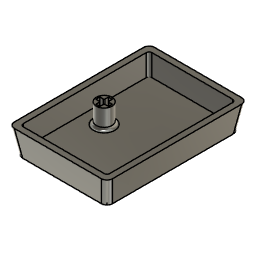
keycaps_tiapad_lcd_f1_f4 (Autodesk Fusion 360 design; units mm, degrees)
Autodesk Fusion 360 part; units mm, degrees
sketch "Schizzo1" plane through (0, 0, 0) normal (0, 0, 1) x (1, 0, 0) in component "keycap"
  circle A0 centre (0, 0) radius 2.8
  line L0 (2.25, 2.25) -> (-2.25, 2.25) construction
  line L1 (-2.25, 2.25) -> (-2.25, -2.25) construction
  line L2 (-2.25, -2.25) -> (2.25, -2.25) construction
  line L3 (2.25, -2.25) -> (2.25, 2.25) construction
  line L4 (2.25, 2.25) -> (-2.25, -2.25) construction
  line L5 (-2.25, 2.25) -> (2.25, -2.25) construction
  line L6 (0.685, 2.2283) -> (-0.685, 2.2283)
  line L7 (-0.685, 2.2283) -> (-0.685, -2.2283)
  line L8 (-0.685, -2.2283) -> (0.685, -2.2283)
  line L9 (0.685, -2.2283) -> (0.685, 2.2283)
  line L10 (0.685, 2.2283) -> (-0.685, -2.2283) construction
  line L11 (-0.685, 2.2283) -> (0.685, -2.2283) construction
  line L12 (2.2283, 0.685) -> (-2.2283, 0.685)
  line L13 (-2.2283, 0.685) -> (-2.2283, -0.685)
  line L14 (-2.2283, -0.685) -> (2.2283, -0.685)
  line L15 (2.2283, -0.685) -> (2.2283, 0.685)
  line L16 (2.2283, 0.685) -> (-2.2283, -0.685) construction
  line L17 (-2.2283, 0.685) -> (2.2283, -0.685) construction
  dimension "d7" = 5.6
  dimension "d8" = 4.5
  dimension "d9" = 4.5
  dimension "d10" = 1.37
  dimension "d11" = 1.37
  constraint coincident A0.centre origin
  constraint horizontal L0
  constraint perpendicular L0 L1
  constraint parallel L0 L2
  constraint parallel L1 L3
  constraint coincident L4 A0.centre
  constraint coincident L5 A0.centre
  constraint horizontal L6
  constraint perpendicular L6 L7
  constraint parallel L6 L8
  constraint parallel L7 L9
  constraint coincident L10 A0.centre
  constraint coincident L11 A0.centre
  constraint horizontal L12
  constraint perpendicular L12 L13
  constraint parallel L12 L14
  constraint parallel L13 L15
  constraint coincident L16 A0.centre
  constraint coincident L17 A0.centre
  measures "d7" diameter of A0
  measures "d8" distance of L1.end L2.end
  measures "d9" distance of L0.end L1.end
  measures "d10" distance of L7.end L8.end
  measures "d11" distance of L12.end L13.end
extrude "Estrusione1" add sketch "Schizzo1" along normal blind 8.45 makes body 1 in component "keycap"
fillet "Raccordo1" radius 0.3 4 edges at (-0.685, 0.685, 4.225) (0.685, 0.685, 4.225) (0.685, -0.685, 4.225) (-0.685, -0.685, 4.225) on bodies 1 in component "keycap"
sketch "Schizzo6" plane through (0, 0, 0) normal (0, 0, -1) x (1, 0, 0)
  arc A0 (-0.985, 0.685) -> (-0.685, 0.985) centre (-0.985, 0.985) ccw
  line L0 (-0.685, 0.985) -> (-0.685, 2.2283)
  line L1 (-0.685, 2.2283) -> (0.685, 2.2283)
  line L2 (0.685, 2.2283) -> (0.685, 0.985)
  arc A1 (0.685, 0.985) -> (0.985, 0.685) centre (0.985, 0.985) ccw
  line L3 (0.985, 0.685) -> (2.2283, 0.685)
  line L4 (2.2283, 0.685) -> (2.2283, -0.685)
  line L5 (2.2283, -0.685) -> (0.985, -0.685)
  arc A2 (0.985, -0.685) -> (0.685, -0.985) centre (0.985, -0.985) ccw
  line L6 (0.685, -0.985) -> (0.685, -2.2283)
  line L7 (0.685, -2.2283) -> (-0.685, -2.2283)
  line L8 (-0.685, -2.2283) -> (-0.685, -0.985)
  arc A3 (-0.685, -0.985) -> (-0.985, -0.685) centre (-0.985, -0.985) ccw
  line L9 (-0.985, -0.685) -> (-2.2283, -0.685)
  line L10 (-2.2283, -0.685) -> (-2.2283, 0.685)
  line L11 (-2.2283, 0.685) -> (-0.985, 0.685)
  circle A4 centre (0, 0) radius 2.8
  line L12 (-7, -7) -> (7, -7)
  line L13 (7, -7) -> (7, 7)
  line L14 (7, 7) -> (-7, 7)
  line L15 (-7, 7) -> (-7, -7)
  line L16 (-7, -7) -> (7, 7) construction
  line L17 (7, -7) -> (-7, 7) construction
  line L18 (9.1, -9.1) -> (-9.1, -9.1)
  line L19 (-9.1, -9.1) -> (-9.1, 9.1)
  line L20 (-9.1, 9.1) -> (9.1, 9.1)
  line L21 (9.1, 9.1) -> (9.1, -9.1)
  line L22 (9.1, -9.1) -> (-9.1, 9.1) construction
  line L23 (-9.1, -9.1) -> (9.1, 9.1) construction
  line L24 (7.6, 7.6) -> (7.6, -7.6)
  line L25 (7.6, -7.6) -> (-7.6, -7.6)
  line L26 (-7.6, -7.6) -> (-7.6, 7.6)
  line L27 (-7.6, 7.6) -> (7.6, 7.6)
  dimension "d37" = 14
  dimension "d38" = 14
  dimension "d42" = 18.2
  dimension "d43" = 18.2
  dimension "d44" = 1.5
  constraint horizontal L12
  constraint perpendicular L12 L13
  constraint parallel L12 L14
  constraint parallel L13 L15
  constraint coincident L16 A4.centre
  constraint coincident L17 A4.centre
  constraint coincident A4.centre origin
  constraint horizontal L18
  constraint perpendicular L18 L19
  constraint parallel L18 L20
  constraint parallel L19 L21
  constraint coincident L22 A4.centre
  constraint coincident L23 A4.centre
  measures "d37" distance of L13.end L14.end
  measures "d38" distance of L12.end L13.end
  measures "d42" distance of L19.end L20.end
  measures "d43" distance of L18.end L19.end
sketch "Schizzo13" plane through (0, 0, 0) normal (0, 0, -1) x (1, 0, 0)
  arc A0 (-0.985, 0.685) -> (-0.685, 0.985) centre (-0.985, 0.985) ccw
  line L0 (-0.685, 0.985) -> (-0.685, 2.2283)
  line L1 (-0.685, 2.2283) -> (0.685, 2.2283)
  line L2 (0.685, 2.2283) -> (0.685, 0.985)
  arc A1 (0.685, 0.985) -> (0.985, 0.685) centre (0.985, 0.985) ccw
  line L3 (0.985, 0.685) -> (2.2283, 0.685)
  line L4 (2.2283, 0.685) -> (2.2283, -0.685)
  line L5 (2.2283, -0.685) -> (0.985, -0.685)
  arc A2 (0.985, -0.685) -> (0.685, -0.985) centre (0.985, -0.985) ccw
  line L6 (0.685, -0.985) -> (0.685, -2.2283)
  line L7 (0.685, -2.2283) -> (-0.685, -2.2283)
  line L8 (-0.685, -2.2283) -> (-0.685, -0.985)
  arc A3 (-0.685, -0.985) -> (-0.985, -0.685) centre (-0.985, -0.985) ccw
  line L9 (-0.985, -0.685) -> (-2.2283, -0.685)
  line L10 (-2.2283, -0.685) -> (-2.2283, 0.685)
  line L11 (-2.2283, 0.685) -> (-0.985, 0.685)
  circle A4 centre (0, 0) radius 2.8
  line L12 (0, 0) -> (-9, 0) construction
  line L13 (-9, 0) -> (-9, 25) construction
  line L14 (-9, 25) -> (26, 25)
  line L15 (26, 25) -> (26, -25)
  line L16 (26, -25) -> (-9, -25)
  line L17 (-9, -25) -> (-9, 25)
  line L18 (24.5, 23.5) -> (24.5, -23.5)
  line L19 (24.5, -23.5) -> (-7.5, -23.5)
  line L20 (-7.5, -23.5) -> (-7.5, 23.5)
  line L21 (-7.5, 23.5) -> (24.5, 23.5)
  line L22 (23.9, 22.9) -> (23.9, -22.9)
  line L23 (23.9, -22.9) -> (-6.9, -22.9)
  line L24 (-6.9, -22.9) -> (-6.9, 22.9)
  line L25 (-6.9, 22.9) -> (23.9, 22.9)
  dimension "d65" = 9
  dimension "d66" = 25
  dimension "d67" = 35
  dimension "d68" = 50
  dimension "d69" = 1.5
  dimension "d70" = 2.1
  constraint coincident A4.centre L12.start
  constraint parallel L3 L12
  constraint perpendicular L12 L13
  constraint horizontal L14
  constraint vertical L15
  constraint horizontal L16
  constraint vertical L17
  measures "d65" distance of A4.centre L12.end
  measures "d66" distance of L12.end L13.end
  measures "d67" distance of L13.end L14.end
  measures "d68" distance of L13.end L16.end
extrude "Estrusione5" add sketch "Schizzo13" against normal blind 9.2 separate body contours L14 L15 L16 L17 | L18 L19 L20 L21 makes body 2
extrude "Estrusione6" [suppressed]
extrude "Estrusione8" add sketch "Schizzo13" against normal blind 1.5 contours A0 L0 L1 L2 A1 L3 L4 L5 A2 L6 L7 L8 A3 L9 L10 L11 | A4 | L22 L23 L24 L25 bodies 1 in component "keycap"
sketch "Schizzo14" plane through (0, -25, 0) normal (0, -1, 0) x (1, 0, 0)
  line L0 (-9, 0) -> (26, 0)
  line L1 (26, 0) -> (26, 9.2)
  line L2 (26, 9.2) -> (-9, 9.2)
  line L3 (-9, 9.2) -> (-9, 0)
  line L4 (-9, 9.2) -> (-7.5, 0)
  line L5 (26, 9.2) -> (24.5, 0)
  point P0 (-7.5, 0)
  point P1 (24.5, 0)
  constraint coincident L2.end L3.start
  constraint coincident P0 L4.end
  constraint coincident L1.end L2.start
  constraint coincident P1 L5.end
sketch "Schizzo15" plane through (26, 0, 0) normal (1, 0, 0) x (0, 1, 0)
  line L0 (-25, 0) -> (25, 0)
  line L1 (25, 0) -> (25, 9.2)
  line L2 (25, 9.2) -> (-25, 9.2)
  line L3 (-25, 9.2) -> (-25, 0)
  line L4 (-25, 9.2) -> (-23.5, 0)
  line L5 (25, 9.2) -> (23.5, 0)
  point P0 (-23.5, 0)
  point P1 (23.5, 0)
  constraint coincident L2.end L3.start
  constraint coincident P0 L4.end
  constraint coincident L1.end L2.start
  constraint coincident P1 L5.end
extrude "Estrusione7" cut sketch "Schizzo14" against normal through all contours L0 L3 L4 | L0 L1 L5 bodies 2
extrude "Estrusione8'" cut sketch "Schizzo15" against normal through all contours L0 L3 L4 | L0 L1 L5 bodies 2
fillet "Raccordo4" radius 1 1 edges at (-2.6105, -1.0125, 1.5) on bodies 1 in component "keycap"
fillet "Raccordo5" radius 0.5 1 faces at (0.2528, 0.2427, 1.5) on bodies 1 in component "keycap"
fillet "Raccordo4'" radius 1 4 edges at (-6.9, 22.9, 4.6) (23.9, 22.9, 4.6) (23.9, -22.9, 4.6) (-6.9, -22.9, 4.6) on bodies 2
fillet "Raccordo5'" radius 2 4 edges at (25.25, 24.25, 4.6) (-8.25, 24.25, 4.6) (-8.25, -24.25, 4.6) (25.25, -24.25, 4.6) on bodies 2
component "keycap" placed x (1, 0, 0) y (0, 1, 0) z (0, 0, 1) at (0, 0, 0)
component "keycap_1" placed x (1, 0, 0) y (0, 1, 0) z (0, 0, 1) at (0, 0, 0)
equation "tol = 0.2 mm"
equation "keystem_height = 3.6 mm"
equation "keystem_cross_lenght = 4.1 mm + tol * 2"
equation "keystem_cross_armwidth = 1.17 mm + tol"
equation "keystem_angle_curvature = 0.3 mm"
equation "shaft_diameter = 5.4 mm + tol"
equation "d7 = shaft_diameter"
equation "d8 = keystem_cross_lenght"
equation "d9 = keystem_cross_lenght"
equation "d10 = keystem_cross_armwidth"
equation "d11 = keystem_cross_armwidth"
equation "d12 = keycap_height - keycap_plasticthickness / 2"
equation "d15 = keystem_angle_curvature"
equation "keycap_side_bottom = 18.2 mm"
equation "keycap_height = 9.2 mm"
equation "keycap_plasticthickness = 1.5 mm"
equation "keycap_side_top = 14 mm"
equation "d37 = keycap_side_top"
equation "d38 = keycap_side_top"
equation "d42 = keycap_side_bottom"
equation "d43 = keycap_side_bottom"
equation "d44 = keycap_plasticthickness"
equation "keycap_f1_f4_side_short = 35 mm"
equation "keycap_f1_f4_side_long = 50 mm"
equation "keycap_f1_f4_dist_from_side_short = 9 mm"
equation "keycap_f1_f4_dist_from_top = keycap_f1_f4_side_long / 2"
equation "d65 = keycap_f1_f4_dist_from_side_short"
equation "d66 = keycap_f1_f4_dist_from_top"
equation "d67 = keycap_f1_f4_side_short"
equation "d68 = keycap_f1_f4_side_long"
equation "d69 = keycap_plasticthickness"
equation "d70 = ( keycap_side_bottom - keycap_side_top ) / 2"
equation "d71 = -keycap_height"
equation "d73 = -keycap_plasticthickness"
equation "d79 = -keycap_plasticthickness"
